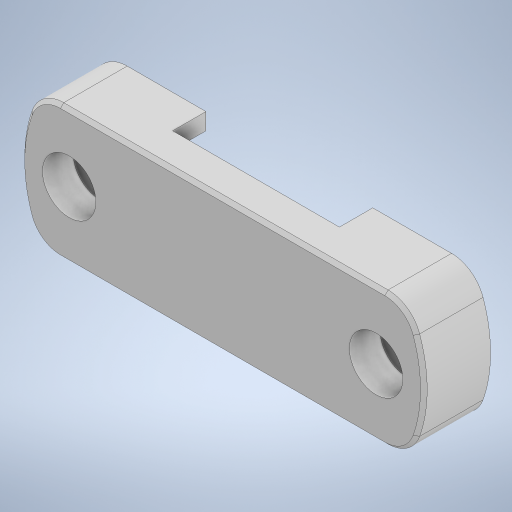
# Autodesk Inventor part: drzak_kable_horni_dil
Saved by Autodesk Inventor 2023 (Build 270158000, 158)
## iProperties
Created: 2025-01-22
Part Number: drzak_kable_horni_dil
Material: Všeobecné
Document SubType Name: Modeling
Designer: lisnik
Density: 1 g/cm^3
Appearance: Výchozí
Author: lisnik
Autodesk Inventor part; units mm, degrees
ref_plane "YZ Plane" through (0, 0, 0) normal (1, 0, 0) x (0, 1, 0)
ref_plane "XZ Plane" through (0, 0, 0) normal (0, 1, 0) x (-1, 0, 0)
ref_plane "XY Plane" through (0, 0, 0) normal (0, 0, 1) x (1, 0, 0)
sketch "Náčrt1" plane through (0, 0, 0) normal (0, 0, 1) x (1, 0, 0)
  line L0 (-24.5, 0) -> (24.5, 0) projected
  line L1 (0, -14) -> (0, 14) projected
  line L2 (-17.5, 10) -> (17.5, 10)
  line L3 (17.5, 10) -> (17.5, -10)
  line L4 (17.5, -10) -> (-17.5, -10)
  line L5 (-17.5, -10) -> (-17.5, 10)
  point P0 (0, 0)
  point P1 (0, 10)
  point P2 (17.5, 0)
  point P3 (-17.5, 0)
  point P4 (0, -10)
  dimension "d0" = 35
  dimension "d1" = 20
  constraints: 8 end point, 2 midpoint, 2 parallel, 2 point on line, 1 horizontal, 1 perpendicular
  measures "d0" distance of L3.end L4.end
  measures "d1" distance of L2.end L3.end
extrude "Vysunutí1" add sketch "Náčrt1" along normal blind 10
sketch "Náčrt2" plane through (0, 0, 0) normal (0, 0, -1) x (-1, 0, 0)
  line L0 (17.5, -10) -> (-17.5, -10) projected
  line L1 (17.5, 10) -> (17.5, -10) projected
  line L2 (-17.5, 10) -> (17.5, 10) projected
  line L3 (-17.5, -10) -> (-17.5, 10) projected
  line L4 (-15, 7.5) -> (15, 7.5)
  line L5 (15, 7.5) -> (15, -7.5)
  line L6 (15, -7.5) -> (-15, -7.5)
  line L7 (-15, -7.5) -> (-15, 7.5)
  line L8 (24.5, 0) -> (-24.5, 0) projected
  line L9 (0, -14) -> (0, 14) projected
  point P0 (0, 0)
  point P1 (0, 7.5)
  point P2 (15, 0)
  dimension "d4" = 15
  dimension "d5" = 30
  constraints: 8 end point, 2 midpoint, 2 parallel, 2 point on line, 1 horizontal, 1 perpendicular
  measures "d4" distance of L4.end L5.end
  measures "d5" distance of L4.start L4.end
extrude "Vysunutí2" cut sketch "Náčrt2" against normal blind 7.5 contours L9 L8 L5 L6 | L6 L7 L8 L9 | L8 L9 L4 L5 | L8 L7 L4 L9
sketch "Náčrt3" plane through (-17.5, 10, 0) normal (0, 1, 0) x (1, 0, 0)
  line L0 (35, 0) -> (0, 0) projected
  line L1 (0, 0) -> (0, -10) projected
  line L2 (35, -10) -> (0, -10) projected
  line L3 (35, 0) -> (35, -10) projected
  line L4 (30, -5) -> (5, -5)
  line L5 (5, -5) -> (5, 0)
  line L6 (5, 0) -> (30, 0)
  line L7 (30, 0) -> (30, -5)
  point P0 (17.5, 0)
  point P1 (17.5, 0)
  point P2 (30, 0)
  point P3 (5, 0)
  dimension "d8" = 5
  dimension "d9" = 25
  constraints: 8 end point, 2 midpoint, 2 parallel, 1 horizontal, 1 perpendicular
  measures "d8" distance of L4.end L5.end
  measures "d9" distance of L4.start L4.end
extrude "Vysunutí3" cut sketch "Náčrt3" against normal through all contours L7 L4 L5 L0
sketch "Náčrt4" plane through (0, 0, 0) normal (0, 0, -1) x (-1, 0, 0)
  line L0 (-12.5, 7.5) -> (-12.5, 10) projected
  line L1 (-17.5, 10) -> (-12.5, 10) projected
  line L2 (-17.5, -10) -> (-17.5, 10) projected
  line L3 (-12.5, -10) -> (-17.5, -10) projected
  line L4 (-12.5, -10) -> (-12.5, -7.5) projected
  line L5 (-12.5, -7.5) -> (-15, -7.5) projected
  line L6 (-15, -7.5) -> (-15, 7.5) projected
  line L7 (-15, 7.5) -> (-12.5, 7.5) projected
  line L8 (12.5, 10) -> (12.5, 7.5) projected
  line L9 (12.5, 7.5) -> (15, 7.5) projected
  line L10 (15, 7.5) -> (15, -7.5) projected
  line L11 (15, -7.5) -> (12.5, -7.5) projected
  line L12 (12.5, -7.5) -> (12.5, -10) projected
  line L13 (17.5, -10) -> (12.5, -10) projected
  line L14 (17.5, 10) -> (17.5, -10) projected
  line L15 (12.5, 10) -> (17.5, 10) projected
  line L16 (52.5, 0) -> (-52.5, 0) projected
  line L17 (0, -14) -> (0, 14) projected
  line L18 (-17.5, 10) -> (17.5, 10) projected
  line L19 (-27.5, 10) -> (-17.5, 10)
  line L20 (-17.5, 10) -> (-17.5, -10)
  line L21 (-17.5, -10) -> (-27.5, -10)
  line L22 (-27.5, -10) -> (-27.5, 10)
  line L23 (17.5, 10) -> (27.5, 10)
  line L24 (27.5, 10) -> (27.5, -10)
  line L25 (27.5, -10) -> (17.5, -10)
  line L26 (17.5, -10) -> (17.5, 10)
  arc A0 (-27.5, 10) -> (-27.5, -10) centre (-10, 0) ccw
  arc A1 (27.5, -10) -> (27.5, 10) centre (10, 0) ccw
  point P0 (0, 0)
  point P1 (-17.5, 0)
  point P2 (17.5, 0)
  point P3 (-17.5, 0)
  point P4 (17.5, 0)
  dimension "d26" = 10
  dimension "d27" = 10
  dimension "d32" = 10
  dimension "d33" = 10
  constraints: 16 end point, 8 point on line, 4 midpoint, 4 parallel, 4 point on circle, 2 centre point, 2 horizontal, 2 perpendicular
  measures "d26" distance of L19.start L19.end
  measures "d27" distance of L23.start L23.end
  measures "d32" distance from line of L17 A0.centre
  measures "d33" distance from line of L17 A1.centre
extrude "Vysunutí4" add sketch "Náčrt4" against normal up to surface (10 mm away) contours L2 L16 L22 L19 | L2 L21 L22 L16 | L22 L16 A0 | L22 A0 L16 | L23 L24 L16 L14 | L16 L24 L25 L14 | A1 L16 L24 | L16 A1 L24
sketch "Náčrt5" plane through (0, 0, 10) normal (0, 0, 1) x (1, 0, 0)
  line L0 (-47.1525, 0) -> (47.1525, 0) projected
  line L1 (0, -14) -> (0, 14) projected
  line L2 (-27.5, 10) -> (27.5, 10) projected
  line L3 (27.5, -10) -> (-27.5, -10) projected
  arc A0 (27.5, -10) -> (27.5, 10) centre (10, 0) ccw projected
  arc A1 (-27.5, 10) -> (-27.5, -10) centre (-10, 0) ccw projected
  point P0 (0, 0)
  point P1 (23, 0)
  point P2 (-23, 0)
  dimension "d30" = 46
  dimension "d31" = 23
  constraints: 2 point on line
  measures "d30" distance of point (-23, 0) point (23, 0)
  measures "d31" distance from line of L1 point (-23, 0)
hole "Díra1" at (23, 0, 10) at (-23, 0, 10) direction (0, 0, -1) diameter 4.5 end through all counterbore diameter 8 counterbore depth 4.6 clearance for "Šroub s hlavou s vnitřním vybráním ISO 4762" size "M4" standard "ISO"
fillet "Zaoblení2" radius 5 4 edges at (27.5, 10, 5) (-27.5, 10, 5) (-27.5, -10, 5) (27.5, -10, 5)
chamfer "Zkosení1" distance 0.5 angle 45 2 edges at (0, 10, 10) (0, -10, 10)
